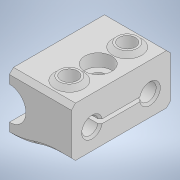
# Autodesk Inventor part: XY Joiner
Saved by Autodesk Inventor 2022 (Build 260153000, 153)
## iProperties
Created: 2022-04-23
Part Number: XY Joiner
Material: Generic
Document SubType Name: Modeling
Designer: Nick
Density: 1 g/cm^3
Appearance: Default
Author: Nick
Autodesk Inventor part; units mm, degrees
ref_plane "YZ Plane" through (0, 0, 0) normal (1, 0, 0) x (0, 1, 0)
ref_plane "XZ Plane" through (0, 0, 0) normal (0, 1, 0) x (-1, 0, 0)
ref_plane "XY Plane" through (0, 0, 0) normal (0, 0, 1) x (1, 0, 0)
sketch "Sketch1" plane through (0, 0, 0) normal (0, 0, 1) x (1, 0, 0)
  line L0 (0, 14) -> (0, 11)
  line L1 (0, 14) -> (15, 14)
  line L2 (15, 14) -> (15, 0)
  circle A0 centre (0, 7) radius 4
  line L3 (0, 3) -> (0, 0)
  line L4 (0, 0) -> (15, 0)
  line L5 (0, 11) -> (0, 3) construction
  dimension "d0" = 8
  dimension "d1" = 15
  dimension "d2" = 14
  constraints: 12 end point, 3 vertical, 2 coincident, 2 horizontal, 1 collinear, 1 midpoint, 1 perpendicular, 3 other
  measures "d1" distance of L0.start L1.end
  measures "d2" distance between parallel lines of L4 L1
extrude "Extrusion1" add sketch "Sketch1" along normal blind 24 contours L1 L2 L4 L3 A0 L0
sketch "Sketch2" plane through (15, 0, 0) normal (1, 0, 0) x (0, 0, -1)
  line L0 (-24, 0) -> (-24, 14) projected
  line L1 (0, 0) -> (0, 14) projected
  point P0 (-19, 7)
  point P1 (-5, 7)
  point P2 (-24, 7)
  dimension "d5" = 5
  dimension "d6" = 5
  dimension "d7" = 14
  constraints: 2 horizontal alignment, 1 midpoint
  measures "d5" distance of point (-24, 7) point (-19, 7)
  measures "d6" distance from line of L1 point (-5, 7)
  measures "d7" distance of point (-5, 7) point (-19, 7)
hole "Hole1" at (15, 7, 19) at (15, 7, 5) direction (-1, 0, 0) diameter 4 depth 8
sketch "Sketch4" plane through (0, 14, 0) normal (0, 1, 0) x (1, 0, 0)
  circle A0 centre (9.5, -5) radius 3.5
  circle A1 centre (9.5, -19) radius 3.5
  line L0 (15, -24) -> (0, -24) projected
  line L1 (15, 0) -> (0, 0) projected
  line L2 (0, 0) -> (0, 0) projected
  line L3 (0, 0) -> (0, -24) projected
  line L4 (0, -24) -> (0, -24) projected
  line L5 (0, 0) -> (0, -24) projected
  line L6 (4, -24) -> (4, 0) projected
  line L7 (4, -24) -> (4, 0)
  line L8 (4, -24) -> (4, 0) projected
  line L9 (15, 0) -> (15, -24) projected
  point P0 (7.5, -24)
  dimension "d18" = 7
  dimension "d19" = 7
  dimension "d20" = 14
  dimension "d21" = 5
  dimension "d22" = 5
  dimension "d42" = 5.5
  dimension "d43" = 5.5
  constraints: 4 point on line, 2 centre point, 2 end point, 1 midpoint, 1 vertical alignment
  measures "d18" diameter of A0
  measures "d19" diameter of A1
  measures "d20" distance of A0.centre A1.centre
  measures "d21" distance from line of L0 A1.centre
  measures "d22" distance from line of A0.centre L1
  measures "d42" distance from line of L6 A1.centre
  measures "d43" distance from line of L9 A1.centre
extrude "Extrusion2" add sketch "Sketch4" along normal blind 1 contours A0 | A1
chamfer "Chamfer1" distance 1 angle 45 2 edges at (6, 15, 19) (6, 15, 5)
sketch "Sketch3" plane through (2, 15, 0) normal (0, 1, 0) x (1, 0, 0)
  line L0 (13, -24) -> (-2, -24) projected
  line L1 (13, 0) -> (-2, 0) projected
  circle A0 centre (7.5, -5) radius 2.5 projected
  circle A1 centre (7.5, -19) radius 2.5 projected
  point P0 (5.5, 0)
  constraints: 2 coincident, 1 midpoint, 1 vertical alignment
hole "Hole2" at (9.5, 15, 19) at (9.5, 15, 5) direction (0, -1, 0) diameter 4 depth 7
sketch "Sketch5" plane through (15, 0, 0) normal (1, 0, 0) x (0, 0, -1)
  line L0 (-17.0635, 7.5) -> (-6.9365, 7.5)
  line L1 (-6.9365, 7.5) -> (-6.9365, 6.5)
  line L2 (-6.9365, 6.5) -> (-17.0635, 6.5)
  line L3 (-17.0635, 6.5) -> (-17.0635, 7.5)
  circle A0 centre (-5, 7) radius 2 projected
  circle A1 centre (-19, 7) radius 2 projected
  point P0 (0, 0)
  point P1 (-6.9365, 7)
  point P2 (-17.0635, 6.5)
  dimension "d35" = 1
  constraints: 8 end point, 2 parallel, 1 horizontal, 1 horizontal alignment, 1 midpoint, 1 perpendicular, 4 other
  measures "d35" distance of L0.end L1.end
extrude "Extrusion3" cut sketch "Sketch5" against normal blind 8 contours L0 A0 L2 A1
sketch "Sketch6" plane through (0, 0, 0) normal (0, 0, -1) x (-1, 0, 0)
  line L0 (0, 3) -> (0, 0) projected
  arc A0 (-6, 1) -> (0, 0) centre (0, 18.5) ccw
  line L1 (-15, 0) -> (-15, 14) projected
  line L2 (-15, 2) -> (-12, 2)
  arc A1 (-6, 1) -> (-12, 2) centre (-12, -16.5) ccw
  line L3 (0, 0) -> (-15, 0) projected
  line L4 (-6, 1) -> (0, 0) construction
  line L5 (-6, 1) -> (-12, 2) construction
  dimension "d38" = 2
  dimension "d39" = 3
  constraints: 6 end point, 4 point on circle, 2 centre point, 2 tangent, 1 collinear, 1 equal radius, 1 horizontal, 1 point on line
  measures "d38" distance between parallel lines of L3 L2
  measures "d39" distance of L2.start L2.end
extrude "Extrusion4" cut sketch "Sketch6" against normal through all
sketch "Sketch7" plane through (0, 14, 0) normal (0, 1, 0) x (1, 0, 0)
  circle A0 centre (9.5, -5) radius 2 projected
  circle A1 centre (9.5, -19) radius 2 projected
  point P0 (0, 0)
  point P1 (9.5, -12)
  dimension "d44" = 7
  dimension "d45" = 7
  constraints: 1 vertical alignment
  measures "d44" distance of A0.centre point (9.5, -12)
  measures "d45" distance of A1.centre point (9.5, -12)
hole "Hole3" at (9.5, 14, 12) direction (0, -1, 0) diameter 3.4 end through all counterbore diameter 6.5 counterbore depth 3 clearance for "Socket Head Cap Screw" size "M3" standard "Ansi Metric M Profile"
chamfer "Chamfer2" distance 1 angle 45 8 edges at (8.9586, 1.7483, 0) (3.0414, 0.2517, 0) (13.5, 2, 0) (7.5, 14, 0) (3.0414, 0.2517, 24) (8.9586, 1.7483, 24) (13.5, 2, 24) (7.5, 14, 24)
chamfer "Chamfer3" distance 0.5 angle 45 2 edges at (15, 7, 3) (15, 7, 21)
sketch "Sketch9" plane through (0, 11, 0) normal (-1, 0, 0) x (0, 0, 1)
  line L0 (2, 2.25) -> (5, 2.25)
  line L1 (5, 2.25) -> (5, 0.75)
  line L2 (5, 0.75) -> (2, 0.75)
  line L3 (2, 0.75) -> (2, 2.25)
  line L4 (7, 2.25) -> (10, 2.25)
  line L5 (10, 2.25) -> (10, 0.75)
  line L6 (10, 0.75) -> (7, 0.75)
  line L7 (7, 0.75) -> (7, 2.25)
  line L8 (14, 2.25) -> (17, 2.25)
  line L9 (17, 2.25) -> (17, 0.75)
  line L10 (17, 0.75) -> (14, 0.75)
  line L11 (14, 0.75) -> (14, 2.25)
  line L12 (19, 2.25) -> (22, 2.25)
  line L13 (22, 2.25) -> (22, 0.75)
  line L14 (22, 0.75) -> (19, 0.75)
  line L15 (19, 0.75) -> (19, 2.25)
  line L16 (1, 3) -> (0, 2) construction
  line L17 (1, 3) -> (1, 0) construction
  line L18 (0, 0) -> (24, 0) construction
  line L19 (12, 0) -> (12, 3) construction
  line L20 (1, 3) -> (23, 3) construction
  line L21 (24, 2) -> (24, 0) construction
  line L22 (0, 2) -> (0, 0) construction
  line L23 (0, 0) -> (0, -8) projected
  line L24 (0, -8) -> (24, -8) projected
  line L25 (24, 0) -> (24, -8) projected
  line L26 (0, 0) -> (24, 0) projected
  line L27 (0, -8) -> (0, 2) construction
  line L28 (0, -4) -> (24, -4) construction
  line L29 (24, -8) -> (24, 2) construction
  point P0 (0, -11)
  point P1 (22, 1.5)
  point P2 (17, 1.5)
  point P3 (14, 1.5)
  point P4 (10, 1.5)
  point P5 (7, 1.5)
  point P6 (5, 1.5)
  point P7 (2, 1.5)
  point P8 (1, 1.5)
  dimension "d65" = 1.5
  dimension "d66" = 3
  dimension "d67" = 2
  dimension "d68" = 2
  dimension "d69" = 2
  dimension "d70" = 2
  dimension "d71" = 2
  dimension "d72" = 2
  constraints: 38 end point, 10 midpoint, 8 parallel, 6 equal length, 5 perpendicular, 4 horizontal, 4 horizontal alignment, 4 point on line, 1 vertical
  measures "d65" distance of L0.end L1.end
  measures "d66" distance of L0.start L0.end
  measures "d67" distance between parallel lines of L11 L19
  measures "d68" distance between parallel lines of L19 L5
  measures "d69" distance between parallel lines of L21 L13
  measures "d70" distance between parallel lines of L22 L3
  measures "d71" distance between parallel lines of L15 L9
  measures "d72" distance between parallel lines of L7 L1
revolve "Revolution1" cut sketch "Sketch9" angle 360 about axis through (0, 7, 0) along (0, 0, 1) contours L0 L1 L2 L3 | L4 L5 L6 L7 | L8 L9 L10 L11 | L12 L13 L14 L15
ref_plane "Work Plane1" through (7, 3.5, 17.0635) normal (0, 1, 0) x (1, 0, 0)
sketch "Sketch10" plane through (7, 3.5, 17.0635) normal (0, 1, 0) x (1, 0, 0)
  circle A0 centre (2.5, 5.0635) radius 1.7 projected
  line L0 (-0.25, 3.4758) -> (-0.25, 6.6512)
  line L1 (-0.25, 6.6512) -> (2.5, 8.2389)
  line L2 (2.5, 8.2389) -> (5.25, 6.6512)
  line L3 (5.25, 6.6512) -> (5.25, 3.4758)
  line L4 (5.25, 3.4758) -> (2.5, 1.8881)
  line L5 (2.5, 1.8881) -> (-0.25, 3.4758)
  point P0 (-7, 17.0635)
  dimension "d75" = 5.5
  constraints: 12 end point, 1 coincident, 1 vertical, 13 other
  measures "d75" distance between parallel lines of L3 L0
extrude "Extrusion6" cut sketch "Sketch10" against normal blind 10
equation "\"d6\" = d5"
equation "\"d22\" = d21"
equation "\"d42\" = d43"
equation "\"d44\" = d45"
equation "\"d68\" = d70"
equation "\"d70\" = d69"
equation "\"d72\" = d71"
body "Solid1"
